Autodesk Fusion 360 part; units mm, degrees
(part 3 of 4)
sketch "草图5" plane through (-64, 0, 0) normal (-1, 0, 0) x (0, -1, 0)
  line L0 (-85, 0) -> (90, 0)
  line L1 (90, 0) -> (90, 250)
  line L2 (90, 250) -> (-85, 250)
  line L3 (-85, 250) -> (-85, 0)
  line L4 (76, 24) -> (67.3397, 19)
  line L5 (67.3397, 19) -> (67.3397, 9)
  line L6 (67.3397, 9) -> (76, 4)
  line L7 (76, 4) -> (84.6603, 9)
  line L8 (84.6603, 9) -> (84.6603, 19)
  line L9 (84.6603, 19) -> (76, 24)
  line L10 (56.6795, 24) -> (48.0192, 19)
  line L11 (48.0192, 19) -> (48.0192, 9)
  line L12 (48.0192, 9) -> (56.6795, 4)
  line L13 (56.6795, 4) -> (65.3397, 9)
  line L14 (65.3397, 9) -> (65.3397, 19)
  line L15 (65.3397, 19) -> (56.6795, 24)
  line L16 (37.359, 24) -> (28.6987, 19)
  line L17 (28.6987, 19) -> (28.6987, 9)
  line L18 (28.6987, 9) -> (37.359, 4)
  line L19 (37.359, 4) -> (46.0192, 9)
  line L20 (46.0192, 9) -> (46.0192, 19)
  line L21 (46.0192, 19) -> (37.359, 24)
  line L22 (18.0385, 24) -> (9.3782, 19)
  line L23 (9.3782, 19) -> (9.3782, 9)
  line L24 (9.3782, 9) -> (18.0385, 4)
  line L25 (18.0385, 4) -> (26.6987, 9)
  line L26 (26.6987, 9) -> (26.6987, 19)
  line L27 (26.6987, 19) -> (18.0385, 24)
  line L28 (-1.282, 24) -> (-9.9423, 19)
  line L29 (-9.9423, 19) -> (-9.9423, 9)
  line L30 (-9.9423, 9) -> (-1.282, 4)
  line L31 (-1.282, 4) -> (7.3782, 9)
  line L32 (7.3782, 9) -> (7.3782, 19)
  line L33 (7.3782, 19) -> (-1.282, 24)
  line L34 (-20.6025, 24) -> (-29.2628, 19)
  line L35 (-29.2628, 19) -> (-29.2628, 9)
  line L36 (-29.2628, 9) -> (-20.6025, 4)
  line L37 (-20.6025, 4) -> (-11.9423, 9)
  line L38 (-11.9423, 9) -> (-11.9423, 19)
  line L39 (-11.9423, 19) -> (-20.6025, 24)
  line L40 (-39.923, 24) -> (-48.5833, 19)
  line L41 (-48.5833, 19) -> (-48.5833, 9)
  line L42 (-48.5833, 9) -> (-39.923, 4)
  line L43 (-39.923, 4) -> (-31.2628, 9)
  line L44 (-31.2628, 9) -> (-31.2628, 19)
  line L45 (-31.2628, 19) -> (-39.923, 24)
  line L46 (-59.2436, 24) -> (-67.9038, 19)
  line L47 (-67.9038, 19) -> (-67.9038, 9)
  line L48 (-67.9038, 9) -> (-59.2436, 4)
  line L49 (-59.2436, 4) -> (-50.5833, 9)
  line L50 (-50.5833, 9) -> (-50.5833, 19)
  line L51 (-50.5833, 19) -> (-59.2436, 24)
  line L52 (66.3397, 40.7321) -> (57.6795, 35.7321)
  line L53 (57.6795, 35.7321) -> (57.6795, 25.7321)
  line L54 (57.6795, 25.7321) -> (66.3397, 20.7321)
  line L55 (66.3397, 20.7321) -> (75, 25.7321)
  line L56 (75, 25.7321) -> (75, 35.7321)
  line L57 (75, 35.7321) -> (66.3397, 40.7321)
  line L58 (47.0192, 40.7321) -> (38.359, 35.7321)
  line L59 (38.359, 35.7321) -> (38.359, 25.7321)
  line L60 (38.359, 25.7321) -> (47.0192, 20.7321)
  line L61 (47.0192, 20.7321) -> (55.6795, 25.7321)
  line L62 (55.6795, 25.7321) -> (55.6795, 35.7321)
  line L63 (55.6795, 35.7321) -> (47.0192, 40.7321)
  line L64 (27.6987, 40.7321) -> (19.0385, 35.7321)
  line L65 (19.0385, 35.7321) -> (19.0385, 25.7321)
  line L66 (19.0385, 25.7321) -> (27.6987, 20.7321)
  line L67 (27.6987, 20.7321) -> (36.359, 25.7321)
  line L68 (36.359, 25.7321) -> (36.359, 35.7321)
  line L69 (36.359, 35.7321) -> (27.6987, 40.7321)
  line L70 (8.3782, 40.7321) -> (-0.282, 35.7321)
  line L71 (-0.282, 35.7321) -> (-0.282, 25.7321)
  line L72 (-0.282, 25.7321) -> (8.3782, 20.7321)
  line L73 (8.3782, 20.7321) -> (17.0385, 25.7321)
  line L74 (17.0385, 25.7321) -> (17.0385, 35.7321)
  line L75 (17.0385, 35.7321) -> (8.3782, 40.7321)
  line L76 (-10.9423, 40.7321) -> (-19.6025, 35.7321)
  line L77 (-19.6025, 35.7321) -> (-19.6025, 25.7321)
  line L78 (-19.6025, 25.7321) -> (-10.9423, 20.7321)
  line L79 (-10.9423, 20.7321) -> (-2.282, 25.7321)
  line L80 (-2.282, 25.7321) -> (-2.282, 35.7321)
  line L81 (-2.282, 35.7321) -> (-10.9423, 40.7321)
  line L82 (-30.2628, 40.7321) -> (-38.923, 35.7321)
  line L83 (-38.923, 35.7321) -> (-38.923, 25.7321)
  line L84 (-38.923, 25.7321) -> (-30.2628, 20.7321)
  line L85 (-30.2628, 20.7321) -> (-21.6025, 25.7321)
  line L86 (-21.6025, 25.7321) -> (-21.6025, 35.7321)
  line L87 (-21.6025, 35.7321) -> (-30.2628, 40.7321)
  line L88 (-49.5833, 40.7321) -> (-58.2436, 35.7321)
  line L89 (-58.2436, 35.7321) -> (-58.2436, 25.7321)
  line L90 (-58.2436, 25.7321) -> (-49.5833, 20.7321)
  line L91 (-49.5833, 20.7321) -> (-40.923, 25.7321)
  line L92 (-40.923, 25.7321) -> (-40.923, 35.7321)
  line L93 (-40.923, 35.7321) -> (-49.5833, 40.7321)
  line L94 (-68.9038, 40.7321) -> (-77.5641, 35.7321)
  line L95 (-77.5641, 35.7321) -> (-77.5641, 25.7321)
  line L96 (-77.5641, 25.7321) -> (-68.9038, 20.7321)
  line L97 (-68.9038, 20.7321) -> (-60.2436, 25.7321)
  line L98 (-60.2436, 25.7321) -> (-60.2436, 35.7321)
  line L99 (-60.2436, 35.7321) -> (-68.9038, 40.7321)
  line L100 (76, 57.4641) -> (67.3397, 52.4641)
  line L101 (67.3397, 52.4641) -> (67.3397, 42.4641)
  line L102 (67.3397, 42.4641) -> (76, 37.4641)
  line L103 (76, 37.4641) -> (84.6603, 42.4641)
  line L104 (84.6603, 42.4641) -> (84.6603, 52.4641)
  line L105 (84.6603, 52.4641) -> (76, 57.4641)
  line L106 (56.6795, 57.4641) -> (48.0192, 52.4641)
  line L107 (48.0192, 52.4641) -> (48.0192, 42.4641)
  line L108 (48.0192, 42.4641) -> (56.6795, 37.4641)
  line L109 (56.6795, 37.4641) -> (65.3397, 42.4641)
  line L110 (65.3397, 42.4641) -> (65.3397, 52.4641)
  line L111 (65.3397, 52.4641) -> (56.6795, 57.4641)
  line L112 (37.359, 57.4641) -> (28.6987, 52.4641)
  line L113 (28.6987, 52.4641) -> (28.6987, 42.4641)
  line L114 (28.6987, 42.4641) -> (37.359, 37.4641)
  line L115 (37.359, 37.4641) -> (46.0192, 42.4641)
  line L116 (46.0192, 42.4641) -> (46.0192, 52.4641)
  line L117 (46.0192, 52.4641) -> (37.359, 57.4641)
  line L118 (18.0385, 57.4641) -> (9.3782, 52.4641)
  line L119 (9.3782, 52.4641) -> (9.3782, 42.4641)
  line L120 (9.3782, 42.4641) -> (18.0385, 37.4641)
  line L121 (18.0385, 37.4641) -> (26.6987, 42.4641)
  line L122 (26.6987, 42.4641) -> (26.6987, 52.4641)
  line L123 (26.6987, 52.4641) -> (18.0385, 57.4641)
  line L124 (-1.282, 57.4641) -> (-9.9423, 52.4641)
  line L125 (-9.9423, 52.4641) -> (-9.9423, 42.4641)
  line L126 (-9.9423, 42.4641) -> (-1.282, 37.4641)
  line L127 (-1.282, 37.4641) -> (7.3782, 42.4641)
  line L128 (7.3782, 42.4641) -> (7.3782, 52.4641)
  line L129 (7.3782, 52.4641) -> (-1.282, 57.4641)
  line L130 (-20.6025, 57.4641) -> (-29.2628, 52.4641)
  line L131 (-29.2628, 52.4641) -> (-29.2628, 42.4641)
  line L132 (-29.2628, 42.4641) -> (-20.6025, 37.4641)
  line L133 (-20.6025, 37.4641) -> (-11.9423, 42.4641)
  line L134 (-11.9423, 42.4641) -> (-11.9423, 52.4641)
  line L135 (-11.9423, 52.4641) -> (-20.6025, 57.4641)
  line L136 (-39.923, 57.4641) -> (-48.5833, 52.4641)
  line L137 (-48.5833, 52.4641) -> (-48.5833, 42.4641)
  line L138 (-48.5833, 42.4641) -> (-39.923, 37.4641)
  line L139 (-39.923, 37.4641) -> (-31.2628, 42.4641)
  line L140 (-31.2628, 42.4641) -> (-31.2628, 52.4641)
  line L141 (-31.2628, 52.4641) -> (-39.923, 57.4641)
  line L142 (-59.2436, 57.4641) -> (-67.9038, 52.4641)
  line L143 (-67.9038, 52.4641) -> (-67.9038, 42.4641)
  line L144 (-67.9038, 42.4641) -> (-59.2436, 37.4641)
  line L145 (-59.2436, 37.4641) -> (-50.5833, 42.4641)
  line L146 (-50.5833, 42.4641) -> (-50.5833, 52.4641)
  line L147 (-50.5833, 52.4641) -> (-59.2436, 57.4641)
  line L148 (66.3397, 74.1962) -> (57.6795, 69.1962)
  line L149 (57.6795, 69.1962) -> (57.6795, 59.1962)
  line L150 (57.6795, 59.1962) -> (66.3397, 54.1962)
  line L151 (66.3397, 54.1962) -> (75, 59.1962)
  line L152 (75, 59.1962) -> (75, 69.1962)
  line L153 (75, 69.1962) -> (66.3397, 74.1962)
  line L154 (47.0192, 74.1962) -> (38.359, 69.1962)
  line L155 (38.359, 69.1962) -> (38.359, 59.1962)
  line L156 (38.359, 59.1962) -> (47.0192, 54.1962)
  line L157 (47.0192, 54.1962) -> (55.6795, 59.1962)
  line L158 (55.6795, 59.1962) -> (55.6795, 69.1962)
  line L159 (55.6795, 69.1962) -> (47.0192, 74.1962)
  line L160 (27.6987, 74.1962) -> (19.0385, 69.1962)
  line L161 (19.0385, 69.1962) -> (19.0385, 59.1962)
  line L162 (19.0385, 59.1962) -> (27.6987, 54.1962)
  line L163 (27.6987, 54.1962) -> (36.359, 59.1962)
  line L164 (36.359, 59.1962) -> (36.359, 69.1962)
  line L165 (36.359, 69.1962) -> (27.6987, 74.1962)
  line L166 (8.3782, 74.1962) -> (-0.282, 69.1962)
  line L167 (-0.282, 69.1962) -> (-0.282, 59.1962)
  line L168 (-0.282, 59.1962) -> (8.3782, 54.1962)
  line L169 (8.3782, 54.1962) -> (17.0385, 59.1962)
  line L170 (17.0385, 59.1962) -> (17.0385, 69.1962)
  line L171 (17.0385, 69.1962) -> (8.3782, 74.1962)
  line L172 (-10.9423, 74.1962) -> (-19.6025, 69.1962)
  line L173 (-19.6025, 69.1962) -> (-19.6025, 59.1962)
  line L174 (-19.6025, 59.1962) -> (-10.9423, 54.1962)
  line L175 (-10.9423, 54.1962) -> (-2.282, 59.1962)
  line L176 (-2.282, 59.1962) -> (-2.282, 69.1962)
  line L177 (-2.282, 69.1962) -> (-10.9423, 74.1962)
  line L178 (-30.2628, 74.1962) -> (-38.923, 69.1962)
  line L179 (-38.923, 69.1962) -> (-38.923, 59.1962)
  line L180 (-38.923, 59.1962) -> (-30.2628, 54.1962)
  line L181 (-30.2628, 54.1962) -> (-21.6025, 59.1962)
  line L182 (-21.6025, 59.1962) -> (-21.6025, 69.1962)
  line L183 (-21.6025, 69.1962) -> (-30.2628, 74.1962)
  line L184 (-49.5833, 74.1962) -> (-58.2436, 69.1962)
  line L185 (-58.2436, 69.1962) -> (-58.2436, 59.1962)
  line L186 (-58.2436, 59.1962) -> (-49.5833, 54.1962)
  line L187 (-49.5833, 54.1962) -> (-40.923, 59.1962)
  line L188 (-40.923, 59.1962) -> (-40.923, 69.1962)
  line L189 (-40.923, 69.1962) -> (-49.5833, 74.1962)
  line L190 (-68.9038, 74.1962) -> (-77.5641, 69.1962)
  line L191 (-77.5641, 69.1962) -> (-77.5641, 59.1962)
  line L192 (-77.5641, 59.1962) -> (-68.9038, 54.1962)
  line L193 (-68.9038, 54.1962) -> (-60.2436, 59.1962)
  line L194 (-60.2436, 59.1962) -> (-60.2436, 69.1962)
  line L195 (-60.2436, 69.1962) -> (-68.9038, 74.1962)
  line L196 (76, 90.9282) -> (67.3397, 85.9282)
  line L197 (67.3397, 85.9282) -> (67.3397, 75.9282)
  line L198 (67.3397, 75.9282) -> (76, 70.9282)
  line L199 (76, 70.9282) -> (84.6603, 75.9282)
  line L200 (84.6603, 75.9282) -> (84.6603, 85.9282)
  line L201 (84.6603, 85.9282) -> (76, 90.9282)
  line L202 (56.6795, 90.9282) -> (48.0192, 85.9282)
  line L203 (48.0192, 85.9282) -> (48.0192, 75.9282)
  line L204 (48.0192, 75.9282) -> (56.6795, 70.9282)
  line L205 (56.6795, 70.9282) -> (65.3397, 75.9282)
  line L206 (65.3397, 75.9282) -> (65.3397, 85.9282)
  line L207 (65.3397, 85.9282) -> (56.6795, 90.9282)
  line L208 (37.359, 90.9282) -> (28.6987, 85.9282)
  line L209 (28.6987, 85.9282) -> (28.6987, 75.9282)
  line L210 (28.6987, 75.9282) -> (37.359, 70.9282)
  line L211 (37.359, 70.9282) -> (46.0192, 75.9282)
  line L212 (46.0192, 75.9282) -> (46.0192, 85.9282)
  line L213 (46.0192, 85.9282) -> (37.359, 90.9282)
  line L214 (18.0385, 90.9282) -> (9.3782, 85.9282)
  line L215 (9.3782, 85.9282) -> (9.3782, 75.9282)
  line L216 (9.3782, 75.9282) -> (18.0385, 70.9282)
  line L217 (18.0385, 70.9282) -> (26.6987, 75.9282)
  line L218 (26.6987, 75.9282) -> (26.6987, 85.9282)
  line L219 (26.6987, 85.9282) -> (18.0385, 90.9282)
  line L220 (-1.282, 90.9282) -> (-9.9423, 85.9282)
  line L221 (-9.9423, 85.9282) -> (-9.9423, 75.9282)
  line L222 (-9.9423, 75.9282) -> (-1.282, 70.9282)
  line L223 (-1.282, 70.9282) -> (7.3782, 75.9282)
  line L224 (7.3782, 75.9282) -> (7.3782, 85.9282)
  line L225 (7.3782, 85.9282) -> (-1.282, 90.9282)
  line L226 (-20.6025, 90.9282) -> (-29.2628, 85.9282)
  line L227 (-29.2628, 85.9282) -> (-29.2628, 75.9282)
  line L228 (-29.2628, 75.9282) -> (-20.6025, 70.9282)
  line L229 (-20.6025, 70.9282) -> (-11.9423, 75.9282)
  line L230 (-11.9423, 75.9282) -> (-11.9423, 85.9282)
  line L231 (-11.9423, 85.9282) -> (-20.6025, 90.9282)
  line L232 (-39.923, 90.9282) -> (-48.5833, 85.9282)
  line L233 (-48.5833, 85.9282) -> (-48.5833, 75.9282)
  line L234 (-48.5833, 75.9282) -> (-39.923, 70.9282)
  line L235 (-39.923, 70.9282) -> (-31.2628, 75.9282)
  line L236 (-31.2628, 75.9282) -> (-31.2628, 85.9282)
  line L237 (-31.2628, 85.9282) -> (-39.923, 90.9282)
  line L238 (-59.2436, 90.9282) -> (-67.9038, 85.9282)
  line L239 (-67.9038, 85.9282) -> (-67.9038, 75.9282)
  line L240 (-67.9038, 75.9282) -> (-59.2436, 70.9282)
  line L241 (-59.2436, 70.9282) -> (-50.5833, 75.9282)
  line L242 (-50.5833, 75.9282) -> (-50.5833, 85.9282)
  line L243 (-50.5833, 85.9282) -> (-59.2436, 90.9282)
  line L244 (66.3397, 107.6603) -> (57.6795, 102.6603)
  line L245 (57.6795, 102.6603) -> (57.6795, 92.6603)
  line L246 (57.6795, 92.6603) -> (66.3397, 87.6603)
  line L247 (66.3397, 87.6603) -> (75, 92.6603)
  line L248 (75, 92.6603) -> (75, 102.6603)
  line L249 (75, 102.6603) -> (66.3397, 107.6603)
  line L250 (47.0192, 107.6603) -> (38.359, 102.6603)
  line L251 (38.359, 102.6603) -> (38.359, 92.6603)
  line L252 (38.359, 92.6603) -> (47.0192, 87.6603)
  line L253 (47.0192, 87.6603) -> (55.6795, 92.6603)
  line L254 (55.6795, 92.6603) -> (55.6795, 102.6603)
  line L255 (55.6795, 102.6603) -> (47.0192, 107.6603)
  line L256 (27.6987, 107.6603) -> (19.0385, 102.6603)
  line L257 (19.0385, 102.6603) -> (19.0385, 92.6603)
  line L258 (19.0385, 92.6603) -> (27.6987, 87.6603)
  line L259 (27.6987, 87.6603) -> (36.359, 92.6603)
  line L260 (36.359, 92.6603) -> (36.359, 102.6603)
  line L261 (36.359, 102.6603) -> (27.6987, 107.6603)
  line L262 (8.3782, 107.6603) -> (-0.282, 102.6603)
  line L263 (-0.282, 102.6603) -> (-0.282, 92.6603)
  line L264 (-0.282, 92.6603) -> (8.3782, 87.6603)
  line L265 (8.3782, 87.6603) -> (17.0385, 92.6603)
  line L266 (17.0385, 92.6603) -> (17.0385, 102.6603)
  line L267 (17.0385, 102.6603) -> (8.3782, 107.6603)
  line L268 (-10.9423, 107.6603) -> (-19.6025, 102.6603)
  line L269 (-19.6025, 102.6603) -> (-19.6025, 92.6603)
  line L270 (-19.6025, 92.6603) -> (-10.9423, 87.6603)
  line L271 (-10.9423, 87.6603) -> (-2.282, 92.6603)
  line L272 (-2.282, 92.6603) -> (-2.282, 102.6603)
  line L273 (-2.282, 102.6603) -> (-10.9423, 107.6603)
  line L274 (-30.2628, 107.6603) -> (-38.923, 102.6603)
  line L275 (-38.923, 102.6603) -> (-38.923, 92.6603)
  line L276 (-38.923, 92.6603) -> (-30.2628, 87.6603)
  line L277 (-30.2628, 87.6603) -> (-21.6025, 92.6603)
  line L278 (-21.6025, 92.6603) -> (-21.6025, 102.6603)
  line L279 (-21.6025, 102.6603) -> (-30.2628, 107.6603)
  line L280 (-49.5833, 107.6603) -> (-58.2436, 102.6603)
  line L281 (-58.2436, 102.6603) -> (-58.2436, 92.6603)
  line L282 (-58.2436, 92.6603) -> (-49.5833, 87.6603)
  line L283 (-49.5833, 87.6603) -> (-40.923, 92.6603)
  line L284 (-40.923, 92.6603) -> (-40.923, 102.6603)
  line L285 (-40.923, 102.6603) -> (-49.5833, 107.6603)
  line L286 (-68.9038, 107.6603) -> (-77.5641, 102.6603)
  line L287 (-77.5641, 102.6603) -> (-77.5641, 92.6603)
  line L288 (-77.5641, 92.6603) -> (-68.9038, 87.6603)
  line L289 (-68.9038, 87.6603) -> (-60.2436, 92.6603)
  line L290 (-60.2436, 92.6603) -> (-60.2436, 102.6603)
  line L291 (-60.2436, 102.6603) -> (-68.9038, 107.6603)
  line L292 (76, 124.3923) -> (67.3397, 119.3923)
  line L293 (67.3397, 119.3923) -> (67.3397, 109.3923)
  line L294 (67.3397, 109.3923) -> (76, 104.3923)
  line L295 (76, 104.3923) -> (84.6603, 109.3923)
  line L296 (84.6603, 109.3923) -> (84.6603, 119.3923)
  line L297 (84.6603, 119.3923) -> (76, 124.3923)
  line L298 (56.6795, 124.3923) -> (48.0192, 119.3923)
  line L299 (48.0192, 119.3923) -> (48.0192, 109.3923)
  line L300 (48.0192, 109.3923) -> (56.6795, 104.3923)
  line L301 (56.6795, 104.3923) -> (65.3397, 109.3923)
  line L302 (65.3397, 109.3923) -> (65.3397, 119.3923)
  line L303 (65.3397, 119.3923) -> (56.6795, 124.3923)
  line L304 (37.359, 124.3923) -> (28.6987, 119.3923)
  line L305 (28.6987, 119.3923) -> (28.6987, 109.3923)
  line L306 (28.6987, 109.3923) -> (37.359, 104.3923)
  line L307 (37.359, 104.3923) -> (46.0192, 109.3923)
  line L308 (46.0192, 109.3923) -> (46.0192, 119.3923)
  line L309 (46.0192, 119.3923) -> (37.359, 124.3923)
  line L310 (18.0385, 124.3923) -> (9.3782, 119.3923)
  line L311 (9.3782, 119.3923) -> (9.3782, 109.3923)
  line L312 (9.3782, 109.3923) -> (18.0385, 104.3923)
  line L313 (18.0385, 104.3923) -> (26.6987, 109.3923)
  line L314 (26.6987, 109.3923) -> (26.6987, 119.3923)
  line L315 (26.6987, 119.3923) -> (18.0385, 124.3923)
  line L316 (-1.282, 124.3923) -> (-9.9423, 119.3923)
  line L317 (-9.9423, 119.3923) -> (-9.9423, 109.3923)
  line L318 (-9.9423, 109.3923) -> (-1.282, 104.3923)
  line L319 (-1.282, 104.3923) -> (7.3782, 109.3923)
  line L320 (7.3782, 109.3923) -> (7.3782, 119.3923)
  line L321 (7.3782, 119.3923) -> (-1.282, 124.3923)
  line L322 (-20.6025, 124.3923) -> (-29.2628, 119.3923)
  line L323 (-29.2628, 119.3923) -> (-29.2628, 109.3923)
  line L324 (-29.2628, 109.3923) -> (-20.6025, 104.3923)
  line L325 (-20.6025, 104.3923) -> (-11.9423, 109.3923)
  line L326 (-11.9423, 109.3923) -> (-11.9423, 119.3923)
  line L327 (-11.9423, 119.3923) -> (-20.6025, 124.3923)
  line L328 (-39.923, 124.3923) -> (-48.5833, 119.3923)
  line L329 (-48.5833, 119.3923) -> (-48.5833, 109.3923)
  line L330 (-48.5833, 109.3923) -> (-39.923, 104.3923)
  line L331 (-39.923, 104.3923) -> (-31.2628, 109.3923)
  line L332 (-31.2628, 109.3923) -> (-31.2628, 119.3923)
  line L333 (-31.2628, 119.3923) -> (-39.923, 124.3923)
  line L334 (-59.2436, 124.3923) -> (-67.9038, 119.3923)
  line L335 (-67.9038, 119.3923) -> (-67.9038, 109.3923)
  line L336 (-67.9038, 109.3923) -> (-59.2436, 104.3923)
  line L337 (-59.2436, 104.3923) -> (-50.5833, 109.3923)
  line L338 (-50.5833, 109.3923) -> (-50.5833, 119.3923)
  line L339 (-50.5833, 119.3923) -> (-59.2436, 124.3923)
  line L340 (66.3397, 141.1244) -> (57.6795, 136.1244)
  line L341 (57.6795, 136.1244) -> (57.6795, 126.1244)
  line L342 (57.6795, 126.1244) -> (66.3397, 121.1244)
  line L343 (66.3397, 121.1244) -> (75, 126.1244)
  line L344 (75, 126.1244) -> (75, 136.1244)
  line L345 (75, 136.1244) -> (66.3397, 141.1244)
  line L346 (47.0192, 141.1244) -> (38.359, 136.1244)
  line L347 (38.359, 136.1244) -> (38.359, 126.1244)
  line L348 (38.359, 126.1244) -> (47.0192, 121.1244)
  line L349 (47.0192, 121.1244) -> (55.6795, 126.1244)
  line L350 (55.6795, 126.1244) -> (55.6795, 136.1244)
  line L351 (55.6795, 136.1244) -> (47.0192, 141.1244)
  line L352 (27.6987, 141.1244) -> (19.0385, 136.1244)
  line L353 (19.0385, 136.1244) -> (19.0385, 126.1244)
  line L354 (19.0385, 126.1244) -> (27.6987, 121.1244)
  line L355 (27.6987, 121.1244) -> (36.359, 126.1244)
  line L356 (36.359, 126.1244) -> (36.359, 136.1244)
  line L357 (36.359, 136.1244) -> (27.6987, 141.1244)
  line L358 (8.3782, 141.1244) -> (-0.282, 136.1244)
  line L359 (-0.282, 136.1244) -> (-0.282, 126.1244)
  line L360 (-0.282, 126.1244) -> (8.3782, 121.1244)
  line L361 (8.3782, 121.1244) -> (17.0385, 126.1244)
  line L362 (17.0385, 126.1244) -> (17.0385, 136.1244)
  line L363 (17.0385, 136.1244) -> (8.3782, 141.1244)
  line L364 (-10.9423, 141.1244) -> (-19.6025, 136.1244)
  line L365 (-19.6025, 136.1244) -> (-19.6025, 126.1244)
  line L366 (-19.6025, 126.1244) -> (-10.9423, 121.1244)
  line L367 (-10.9423, 121.1244) -> (-2.282, 126.1244)
  line L368 (-2.282, 126.1244) -> (-2.282, 136.1244)
  line L369 (-2.282, 136.1244) -> (-10.9423, 141.1244)
  line L370 (-30.2628, 141.1244) -> (-38.923, 136.1244)
  line L371 (-38.923, 136.1244) -> (-38.923, 126.1244)
  line L372 (-38.923, 126.1244) -> (-30.2628, 121.1244)
  line L373 (-30.2628, 121.1244) -> (-21.6025, 126.1244)
  line L374 (-21.6025, 126.1244) -> (-21.6025, 136.1244)
  line L375 (-21.6025, 136.1244) -> (-30.2628, 141.1244)
  line L376 (-49.5833, 141.1244) -> (-58.2436, 136.1244)
  line L377 (-58.2436, 136.1244) -> (-58.2436, 126.1244)
  line L378 (-58.2436, 126.1244) -> (-49.5833, 121.1244)
  line L379 (-49.5833, 121.1244) -> (-40.923, 126.1244)
  line L380 (-40.923, 126.1244) -> (-40.923, 136.1244)
  line L381 (-40.923, 136.1244) -> (-49.5833, 141.1244)
  line L382 (-68.9038, 141.1244) -> (-77.5641, 136.1244)
  line L383 (-77.5641, 136.1244) -> (-77.5641, 126.1244)
  line L384 (-77.5641, 126.1244) -> (-68.9038, 121.1244)
  line L385 (-68.9038, 121.1244) -> (-60.2436, 126.1244)
  line L386 (-60.2436, 126.1244) -> (-60.2436, 136.1244)
  line L387 (-60.2436, 136.1244) -> (-68.9038, 141.1244)
  line L388 (76, 157.8564) -> (67.3397, 152.8564)
  line L389 (67.3397, 152.8564) -> (67.3397, 142.8564)
  line L390 (67.3397, 142.8564) -> (76, 137.8564)
  line L391 (76, 137.8564) -> (84.6603, 142.8564)
  line L392 (84.6603, 142.8564) -> (84.6603, 152.8564)
  line L393 (84.6603, 152.8564) -> (76, 157.8564)
  line L394 (56.6795, 157.8564) -> (48.0192, 152.8564)
  line L395 (48.0192, 152.8564) -> (48.0192, 142.8564)
  line L396 (48.0192, 142.8564) -> (56.6795, 137.8564)
  line L397 (56.6795, 137.8564) -> (65.3397, 142.8564)
  line L398 (65.3397, 142.8564) -> (65.3397, 152.8564)
  line L399 (65.3397, 152.8564) -> (56.6795, 157.8564)
  line L400 (37.359, 157.8564) -> (28.6987, 152.8564)
  line L401 (28.6987, 152.8564) -> (28.6987, 142.8564)
  line L402 (28.6987, 142.8564) -> (37.359, 137.8564)
  line L403 (37.359, 137.8564) -> (46.0192, 142.8564)
  line L404 (46.0192, 142.8564) -> (46.0192, 152.8564)
  line L405 (46.0192, 152.8564) -> (37.359, 157.8564)
  line L406 (18.0385, 157.8564) -> (9.3782, 152.8564)
  line L407 (9.3782, 152.8564) -> (9.3782, 142.8564)
  line L408 (9.3782, 142.8564) -> (18.0385, 137.8564)
  line L409 (18.0385, 137.8564) -> (26.6987, 142.8564)
  line L410 (26.6987, 142.8564) -> (26.6987, 152.8564)
  line L411 (26.6987, 152.8564) -> (18.0385, 157.8564)
  line L412 (-1.282, 157.8564) -> (-9.9423, 152.8564)
  line L413 (-9.9423, 152.8564) -> (-9.9423, 142.8564)
  line L414 (-9.9423, 142.8564) -> (-1.282, 137.8564)
  line L415 (-1.282, 137.8564) -> (7.3782, 142.8564)
  line L416 (7.3782, 142.8564) -> (7.3782, 152.8564)
  line L417 (7.3782, 152.8564) -> (-1.282, 157.8564)
  line L418 (-20.6025, 157.8564) -> (-29.2628, 152.8564)
  line L419 (-29.2628, 152.8564) -> (-29.2628, 142.8564)
  line L420 (-29.2628, 142.8564) -> (-20.6025, 137.8564)
  line L421 (-20.6025, 137.8564) -> (-11.9423, 142.8564)
  line L422 (-11.9423, 142.8564) -> (-11.9423, 152.8564)
  line L423 (-11.9423, 152.8564) -> (-20.6025, 157.8564)
  line L424 (-39.923, 157.8564) -> (-48.5833, 152.8564)
  line L425 (-48.5833, 152.8564) -> (-48.5833, 142.8564)
  line L426 (-48.5833, 142.8564) -> (-39.923, 137.8564)
  line L427 (-39.923, 137.8564) -> (-31.2628, 142.8564)
  line L428 (-31.2628, 142.8564) -> (-31.2628, 152.8564)
  line L429 (-31.2628, 152.8564) -> (-39.923, 157.8564)
  line L430 (-59.2436, 157.8564) -> (-67.9038, 152.8564)
  line L431 (-67.9038, 152.8564) -> (-67.9038, 142.8564)
  line L432 (-67.9038, 142.8564) -> (-59.2436, 137.8564)
  line L433 (-59.2436, 137.8564) -> (-50.5833, 142.8564)
  line L434 (-50.5833, 142.8564) -> (-50.5833, 152.8564)
  line L435 (-50.5833, 152.8564) -> (-59.2436, 157.8564)
  line L436 (66.3397, 174.5885) -> (57.6795, 169.5885)
  line L437 (57.6795, 169.5885) -> (57.6795, 159.5885)
  line L438 (57.6795, 159.5885) -> (66.3397, 154.5885)
  line L439 (66.3397, 154.5885) -> (75, 159.5885)
  line L440 (75, 159.5885) -> (75, 169.5885)
  line L441 (75, 169.5885) -> (66.3397, 174.5885)
  line L442 (47.0192, 174.5885) -> (38.359, 169.5885)
  line L443 (38.359, 169.5885) -> (38.359, 159.5885)
  line L444 (38.359, 159.5885) -> (47.0192, 154.5885)
  line L445 (47.0192, 154.5885) -> (55.6795, 159.5885)
  line L446 (55.6795, 159.5885) -> (55.6795, 169.5885)
  line L447 (55.6795, 169.5885) -> (47.0192, 174.5885)
  line L448 (27.6987, 174.5885) -> (19.0385, 169.5885)
  line L449 (19.0385, 169.5885) -> (19.0385, 159.5885)
  line L450 (19.0385, 159.5885) -> (27.6987, 154.5885)
  line L451 (27.6987, 154.5885) -> (36.359, 159.5885)
  line L452 (36.359, 159.5885) -> (36.359, 169.5885)
  line L453 (36.359, 169.5885) -> (27.6987, 174.5885)
  line L454 (8.3782, 174.5885) -> (-0.282, 169.5885)
  line L455 (-0.282, 169.5885) -> (-0.282, 159.5885)
  line L456 (-0.282, 159.5885) -> (8.3782, 154.5885)
  line L457 (8.3782, 154.5885) -> (17.0385, 159.5885)
  line L458 (17.0385, 159.5885) -> (17.0385, 169.5885)
  line L459 (17.0385, 169.5885) -> (8.3782, 174.5885)
  line L460 (-10.9423, 174.5885) -> (-19.6025, 169.5885)
  line L461 (-19.6025, 169.5885) -> (-19.6025, 159.5885)
  line L462 (-19.6025, 159.5885) -> (-10.9423, 154.5885)
  line L463 (-10.9423, 154.5885) -> (-2.282, 159.5885)
  line L464 (-2.282, 159.5885) -> (-2.282, 169.5885)
  line L465 (-2.282, 169.5885) -> (-10.9423, 174.5885)
  line L466 (-30.2628, 174.5885) -> (-38.923, 169.5885)
  line L467 (-38.923, 169.5885) -> (-38.923, 159.5885)
  line L468 (-38.923, 159.5885) -> (-30.2628, 154.5885)
  line L469 (-30.2628, 154.5885) -> (-21.6025, 159.5885)
  line L470 (-21.6025, 159.5885) -> (-21.6025, 169.5885)
  line L471 (-21.6025, 169.5885) -> (-30.2628, 174.5885)
  line L472 (-49.5833, 174.5885) -> (-58.2436, 169.5885)
  line L473 (-58.2436, 169.5885) -> (-58.2436, 159.5885)
  line L474 (-58.2436, 159.5885) -> (-49.5833, 154.5885)
  line L475 (-49.5833, 154.5885) -> (-40.923, 159.5885)
  line L476 (-40.923, 159.5885) -> (-40.923, 169.5885)
  line L477 (-40.923, 169.5885) -> (-49.5833, 174.5885)
  line L478 (-68.9038, 174.5885) -> (-77.5641, 169.5885)
  line L479 (-77.5641, 169.5885) -> (-77.5641, 159.5885)
  line L480 (-77.5641, 159.5885) -> (-68.9038, 154.5885)
  line L481 (-68.9038, 154.5885) -> (-60.2436, 159.5885)
  line L482 (-60.2436, 159.5885) -> (-60.2436, 169.5885)
  line L483 (-60.2436, 169.5885) -> (-68.9038, 174.5885)
  line L484 (76, 191.3205) -> (67.3397, 186.3205)
  line L485 (67.3397, 186.3205) -> (67.3397, 176.3205)
  line L486 (67.3397, 176.3205) -> (76, 171.3205)
  line L487 (76, 171.3205) -> (84.6603, 176.3205)
  line L488 (84.6603, 176.3205) -> (84.6603, 186.3205)
  line L489 (84.6603, 186.3205) -> (76, 191.3205)
  line L490 (56.6795, 191.3205) -> (48.0192, 186.3205)
  line L491 (48.0192, 186.3205) -> (48.0192, 176.3205)
  line L492 (48.0192, 176.3205) -> (56.6795, 171.3205)
  line L493 (56.6795, 171.3205) -> (65.3397, 176.3205)
  line L494 (65.3397, 176.3205) -> (65.3397, 186.3205)
  line L495 (65.3397, 186.3205) -> (56.6795, 191.3205)
  line L496 (37.359, 191.3205) -> (28.6987, 186.3205)
  line L497 (28.6987, 186.3205) -> (28.6987, 176.3205)
  line L498 (28.6987, 176.3205) -> (37.359, 171.3205)
  line L499 (37.359, 171.3205) -> (46.0192, 176.3205)
  line L500 (46.0192, 176.3205) -> (46.0192, 186.3205)
  line L501 (46.0192, 186.3205) -> (37.359, 191.3205)
  line L502 (18.0385, 191.3205) -> (9.3782, 186.3205)
  line L503 (9.3782, 186.3205) -> (9.3782, 176.3205)
  line L504 (9.3782, 176.3205) -> (18.0385, 171.3205)
  line L505 (18.0385, 171.3205) -> (26.6987, 176.3205)
  line L506 (26.6987, 176.3205) -> (26.6987, 186.3205)
  line L507 (26.6987, 186.3205) -> (18.0385, 191.3205)
  line L508 (-1.282, 191.3205) -> (-9.9423, 186.3205)
  line L509 (-9.9423, 186.3205) -> (-9.9423, 176.3205)
  line L510 (-9.9423, 176.3205) -> (-1.282, 171.3205)
  line L511 (-1.282, 171.3205) -> (7.3782, 176.3205)
  line L512 (7.3782, 176.3205) -> (7.3782, 186.3205)
  line L513 (7.3782, 186.3205) -> (-1.282, 191.3205)
  line L514 (-20.6025, 191.3205) -> (-29.2628, 186.3205)
  line L515 (-29.2628, 186.3205) -> (-29.2628, 176.3205)
  line L516 (-29.2628, 176.3205) -> (-20.6025, 171.3205)
  line L517 (-20.6025, 171.3205) -> (-11.9423, 176.3205)
  line L518 (-11.9423, 176.3205) -> (-11.9423, 186.3205)
  line L519 (-11.9423, 186.3205) -> (-20.6025, 191.3205)
  line L520 (-39.923, 191.3205) -> (-48.5833, 186.3205)
  line L521 (-48.5833, 186.3205) -> (-48.5833, 176.3205)
  line L522 (-48.5833, 176.3205) -> (-39.923, 171.3205)
  line L523 (-39.923, 171.3205) -> (-31.2628, 176.3205)
  line L524 (-31.2628, 176.3205) -> (-31.2628, 186.3205)
  line L525 (-31.2628, 186.3205) -> (-39.923, 191.3205)
  line L526 (-59.2436, 191.3205) -> (-67.9038, 186.3205)
  line L527 (-67.9038, 186.3205) -> (-67.9038, 176.3205)
  line L528 (-67.9038, 176.3205) -> (-59.2436, 171.3205)
  line L529 (-59.2436, 171.3205) -> (-50.5833, 176.3205)
  line L530 (-50.5833, 176.3205) -> (-50.5833, 186.3205)
  line L531 (-50.5833, 186.3205) -> (-59.2436, 191.3205)
  line L532 (66.3397, 208.0526) -> (57.6795, 203.0526)
  line L533 (57.6795, 203.0526) -> (57.6795, 193.0526)
  line L534 (57.6795, 193.0526) -> (66.3397, 188.0526)
  line L535 (66.3397, 188.0526) -> (75, 193.0526)
  line L536 (75, 193.0526) -> (75, 203.0526)
  line L537 (75, 203.0526) -> (66.3397, 208.0526)
  line L538 (47.0192, 208.0526) -> (38.359, 203.0526)
  line L539 (38.359, 203.0526) -> (38.359, 193.0526)
  line L540 (38.359, 193.0526) -> (47.0192, 188.0526)
  line L541 (47.0192, 188.0526) -> (55.6795, 193.0526)
  line L542 (55.6795, 193.0526) -> (55.6795, 203.0526)
  line L543 (55.6795, 203.0526) -> (47.0192, 208.0526)
  line L544 (27.6987, 208.0526) -> (19.0385, 203.0526)
  line L545 (19.0385, 203.0526) -> (19.0385, 193.0526)
  line L546 (19.0385, 193.0526) -> (27.6987, 188.0526)
  line L547 (27.6987, 188.0526) -> (36.359, 193.0526)
  line L548 (36.359, 193.0526) -> (36.359, 203.0526)
  line L549 (36.359, 203.0526) -> (27.6987, 208.0526)
  line L550 (8.3782, 208.0526) -> (-0.282, 203.0526)
  line L551 (-0.282, 203.0526) -> (-0.282, 193.0526)
  line L552 (-0.282, 193.0526) -> (8.3782, 188.0526)
  line L553 (8.3782, 188.0526) -> (17.0385, 193.0526)
  line L554 (17.0385, 193.0526) -> (17.0385, 203.0526)
  line L555 (17.0385, 203.0526) -> (8.3782, 208.0526)
  line L556 (-10.9423, 208.0526) -> (-19.6025, 203.0526)
  line L557 (-19.6025, 203.0526) -> (-19.6025, 193.0526)
  line L558 (-19.6025, 193.0526) -> (-10.9423, 188.0526)
  line L559 (-10.9423, 188.0526) -> (-2.282, 193.0526)
  line L560 (-2.282, 193.0526) -> (-2.282, 203.0526)
  line L561 (-2.282, 203.0526) -> (-10.9423, 208.0526)
  line L562 (-30.2628, 208.0526) -> (-38.923, 203.0526)
  line L563 (-38.923, 203.0526) -> (-38.923, 193.0526)
  line L564 (-38.923, 193.0526) -> (-30.2628, 188.0526)
  line L565 (-30.2628, 188.0526) -> (-21.6025, 193.0526)
  line L566 (-21.6025, 193.0526) -> (-21.6025, 203.0526)
  line L567 (-21.6025, 203.0526) -> (-30.2628, 208.0526)
  line L568 (-49.5833, 208.0526) -> (-58.2436, 203.0526)
  line L569 (-58.2436, 203.0526) -> (-58.2436, 193.0526)
  line L570 (-58.2436, 193.0526) -> (-49.5833, 188.0526)
  line L571 (-49.5833, 188.0526) -> (-40.923, 193.0526)
  line L572 (-40.923, 193.0526) -> (-40.923, 203.0526)
  line L573 (-40.923, 203.0526) -> (-49.5833, 208.0526)
  line L574 (-68.9038, 208.0526) -> (-77.5641, 203.0526)
  line L575 (-77.5641, 203.0526) -> (-77.5641, 193.0526)
  line L576 (-77.5641, 193.0526) -> (-68.9038, 188.0526)
  line L577 (-68.9038, 188.0526) -> (-60.2436, 193.0526)
  line L578 (-60.2436, 193.0526) -> (-60.2436, 203.0526)
  line L579 (-60.2436, 203.0526) -> (-68.9038, 208.0526)
  line L580 (76, 224.7846) -> (67.3397, 219.7846)
  line L581 (67.3397, 219.7846) -> (67.3397, 209.7846)
  line L582 (67.3397, 209.7846) -> (76, 204.7846)
  line L583 (76, 204.7846) -> (84.6603, 209.7846)
  line L584 (84.6603, 209.7846) -> (84.6603, 219.7846)
  line L585 (84.6603, 219.7846) -> (76, 224.7846)
  line L586 (56.6795, 224.7846) -> (48.0192, 219.7846)
  line L587 (48.0192, 219.7846) -> (48.0192, 209.7846)
  line L588 (48.0192, 209.7846) -> (56.6795, 204.7846)
  line L589 (56.6795, 204.7846) -> (65.3397, 209.7846)
  line L590 (65.3397, 209.7846) -> (65.3397, 219.7846)
  line L591 (65.3397, 219.7846) -> (56.6795, 224.7846)
  line L592 (37.359, 224.7846) -> (28.6987, 219.7846)
  line L593 (28.6987, 219.7846) -> (28.6987, 209.7846)
  line L594 (28.6987, 209.7846) -> (37.359, 204.7846)
  line L595 (37.359, 204.7846) -> (46.0192, 209.7846)
  line L596 (46.0192, 209.7846) -> (46.0192, 219.7846)
  line L597 (46.0192, 219.7846) -> (37.359, 224.7846)
  line L598 (18.0385, 224.7846) -> (9.3782, 219.7846)
  line L599 (9.3782, 219.7846) -> (9.3782, 209.7846)
  line L600 (9.3782, 209.7846) -> (18.0385, 204.7846)
  line L601 (18.0385, 204.7846) -> (26.6987, 209.7846)
  line L602 (26.6987, 209.7846) -> (26.6987, 219.7846)
  line L603 (26.6987, 219.7846) -> (18.0385, 224.7846)
  line L604 (-1.282, 224.7846) -> (-9.9423, 219.7846)
  line L605 (-9.9423, 219.7846) -> (-9.9423, 209.7846)
  line L606 (-9.9423, 209.7846) -> (-1.282, 204.7846)
  line L607 (-1.282, 204.7846) -> (7.3782, 209.7846)
  line L608 (7.3782, 209.7846) -> (7.3782, 219.7846)
  line L609 (7.3782, 219.7846) -> (-1.282, 224.7846)
  line L610 (-20.6025, 224.7846) -> (-29.2628, 219.7846)
  line L611 (-29.2628, 219.7846) -> (-29.2628, 209.7846)
  line L612 (-29.2628, 209.7846) -> (-20.6025, 204.7846)
  line L613 (-20.6025, 204.7846) -> (-11.9423, 209.7846)
  line L614 (-11.9423, 209.7846) -> (-11.9423, 219.7846)
  line L615 (-11.9423, 219.7846) -> (-20.6025, 224.7846)
  line L616 (-39.923, 224.7846) -> (-48.5833, 219.7846)
  line L617 (-48.5833, 219.7846) -> (-48.5833, 209.7846)
  line L618 (-48.5833, 209.7846) -> (-39.923, 204.7846)
  line L619 (-39.923, 204.7846) -> (-31.2628, 209.7846)
  line L620 (-31.2628, 209.7846) -> (-31.2628, 219.7846)
  line L621 (-31.2628, 219.7846) -> (-39.923, 224.7846)
  line L622 (-59.2436, 224.7846) -> (-67.9038, 219.7846)
  line L623 (-67.9038, 219.7846) -> (-67.9038, 209.7846)
  line L624 (-67.9038, 209.7846) -> (-59.2436, 204.7846)
  line L625 (-59.2436, 204.7846) -> (-50.5833, 209.7846)
  line L626 (-50.5833, 209.7846) -> (-50.5833, 219.7846)
  line L627 (-50.5833, 219.7846) -> (-59.2436, 224.7846)
  line L628 (66.3397, 241.5167) -> (57.6795, 236.5167)
  line L629 (57.6795, 236.5167) -> (57.6795, 226.5167)
  line L630 (57.6795, 226.5167) -> (66.3397, 221.5167)
  line L631 (66.3397, 221.5167) -> (75, 226.5167)
  line L632 (75, 226.5167) -> (75, 236.5167)
  line L633 (75, 236.5167) -> (66.3397, 241.5167)
  line L634 (47.0192, 241.5167) -> (38.359, 236.5167)
  line L635 (38.359, 236.5167) -> (38.359, 226.5167)
  line L636 (38.359, 226.5167) -> (47.0192, 221.5167)
  line L637 (47.0192, 221.5167) -> (55.6795, 226.5167)
  line L638 (55.6795, 226.5167) -> (55.6795, 236.5167)
  line L639 (55.6795, 236.5167) -> (47.0192, 241.5167)
  line L640 (27.6987, 241.5167) -> (19.0385, 236.5167)
  line L641 (19.0385, 236.5167) -> (19.0385, 226.5167)
  line L642 (19.0385, 226.5167) -> (27.6987, 221.5167)
  line L643 (27.6987, 221.5167) -> (36.359, 226.5167)
  line L644 (36.359, 226.5167) -> (36.359, 236.5167)
  line L645 (36.359, 236.5167) -> (27.6987, 241.5167)
  line L646 (8.3782, 241.5167) -> (-0.282, 236.5167)
  line L647 (-0.282, 236.5167) -> (-0.282, 226.5167)
  line L648 (-0.282, 226.5167) -> (8.3782, 221.5167)
  line L649 (8.3782, 221.5167) -> (17.0385, 226.5167)
  line L650 (17.0385, 226.5167) -> (17.0385, 236.5167)
  line L651 (17.0385, 236.5167) -> (8.3782, 241.5167)
  line L652 (-10.9423, 241.5167) -> (-19.6025, 236.5167)
  line L653 (-19.6025, 236.5167) -> (-19.6025, 226.5167)
  line L654 (-19.6025, 226.5167) -> (-10.9423, 221.5167)
  line L655 (-10.9423, 221.5167) -> (-2.282, 226.5167)
  line L656 (-2.282, 226.5167) -> (-2.282, 236.5167)
  line L657 (-2.282, 236.5167) -> (-10.9423, 241.5167)
  line L658 (-30.2628, 241.5167) -> (-38.923, 236.5167)
  line L659 (-38.923, 236.5167) -> (-38.923, 226.5167)
  line L660 (-38.923, 226.5167) -> (-30.2628, 221.5167)
  line L661 (-30.2628, 221.5167) -> (-21.6025, 226.5167)
  line L662 (-21.6025, 226.5167) -> (-21.6025, 236.5167)
  line L663 (-21.6025, 236.5167) -> (-30.2628, 241.5167)
  line L664 (-49.5833, 241.5167) -> (-58.2436, 236.5167)
  line L665 (-58.2436, 236.5167) -> (-58.2436, 226.5167)
  line L666 (-58.2436, 226.5167) -> (-49.5833, 221.5167)
  line L667 (-49.5833, 221.5167) -> (-40.923, 226.5167)
  line L668 (-40.923, 226.5167) -> (-40.923, 236.5167)
  line L669 (-40.923, 236.5167) -> (-49.5833, 241.5167)
  line L670 (-68.9038, 241.5167) -> (-77.5641, 236.5167)
  line L671 (-77.5641, 236.5167) -> (-77.5641, 226.5167)
  line L672 (-77.5641, 226.5167) -> (-68.9038, 221.5167)
  line L673 (-68.9038, 221.5167) -> (-60.2436, 226.5167)
  line L674 (-60.2436, 226.5167) -> (-60.2436, 236.5167)
  line L675 (-60.2436, 236.5167) -> (-68.9038, 241.5167)
extrude "拉伸5" cut sketch "草图5" against normal blind 4 contours L4 L5 L6 L7 L8 L9 | L10 L11 L12 L13 L14 L15 | L16 L17 L18 L19 L20 L21 | L22 L23 L24 L25 L26 L27 | L28 L29 L30 L31 L32 L33 | L34 L35 L36 L37 L38 L39 | L40 L41 L42 L43 L44 L45 | L46 L47 L48 L49 L50 L51 | L52 L53 L54 L55 L56 L57 | L58 L59 L60 L61 L62 L63 | L64 L65 L66 L67 L68 L69 | L70 L71 L72 L73 L74 L75 | L76 L77 L78 L79 L80 L81 | L82 L83 L84 L85 L86 L87 | L88 L89 L90 L91 L92 L93 | L94 L95 L96 L97 L98 L99 | L100 L101 L102 L103 L104 L105 | L106 L107 L108 L109 L110 L111 | L112 L113 L114 L115 L116 L117 | L118 L119 L120 L121 L122 L123 | L124 L125 L126 L127 L128 L129 | L130 L131 L132 L133 L134 L135 | L136 L137 L138 L139 L140 L141 | L142 L143 L144 L145 L146 L147 | L148 L149 L150 L151 L152 L153 | L154 L155 L156 L157 L158 L159 | L160 L161 L162 L163 L164 L165 | L166 L167 L168 L169 L170 L171 | L172 L173 L174 L175 L176 L177 | L178 L179 L180 L181 L182 L183 | L184 L185 L186 L187 L188 L189 | L190 L191 L192 L193 L194 L195 | L196 L197 L198 L199 L200 L201 | L202 L203 L204 L205 L206 L207 | L208 L209 L210 L211 L212 L213 | L214 L215 L216 L217 L218 L219 | L220 L221 L222 L223 L224 L225 | L226 L227 L228 L229 L230 L231 | L232 L233 L234 L235 L236 L237 | L238 L239 L240 L241 L242 L243 | L244 L245 L246 L247 L248 L249 | L250 L251 L252 L253 L254 L255 | L256 L257 L258 L259 L260 L261 | L262 L263 L264 L265 L266 L267 | L268 L269 L270 L271 L272 L273 | L274 L275 L276 L277 L278 L279 | L280 L281 L282 L283 L284 L285 | L286 L287 L288 L289 L290 L291 | L292 L293 L294 L295 L296 L297 | L298 L299 L300 L301 L302 L303 | L304 L305 L306 L307 L308 L309 | L310 L311 L312 L313 L314 L315 | L316 L317 L318 L319 L320 L321 | L322 L323 L324 L325 L326 L327 | L328 L329 L330 L331 L332 L333 | L334 L335 L336 L337 L338 L339 | L340 L341 L342 L343 L344 L345 | L346 L347 L348 L349 L350 L351 | L352 L353 L354 L355 L356 L357 | L358 L359 L360 L361 L362 L363 | L364 L365 L366 L367 L368 L369 | L370 L371 L372 L373 L374 L375 | L376 L377 L378 L379 L380 L381 | L382 L383 L384 L385 L386 L387 | L388 L389 L390 L391 L392 L393 | L394 L395 L396 L397 L398 L399 | L400 L401 L402 L403 L404 L405 | L406 L407 L408 L409 L410 L411 | L412 L413 L414 L415 L416 L417 | L418 L419 L420 L421 L422 L423 | L424 L425 L426 L427 L428 L429 | L430 L431 L432 L433 L434 L435 | L436 L437 L438 L439 L440 L441 | L442 L443 L444 L445 L446 L447 | L448 L449 L450 L451 L452 L453 | L454 L455 L456 L457 L458 L459 | L460 L461 L462 L463 L464 L465 | L466 L467 L468 L469 L470 L471 | L472 L473 L474 L475 L476 L477 | L478 L479 L480 L481 L482 L483 | L484 L485 L486 L487 L488 L489 | L490 L491 L492 L493 L494 L495 | L496 L497 L498 L499 L500 L501 | L502 L503 L504 L505 L506 L507 | L508 L509 L510 L511 L512 L513 | L514 L515 L516 L517 L518 L519 | L520 L521 L522 L523 L524 L525 | L526 L527 L528 L529 L530 L531 | L532 L533 L534 L535 L536 L537 | L538 L539 L540 L541 L542 L543 | L544 L545 L546 L547 L548 L549 | L550 L551 L552 L553 L554 L555 | L556 L557 L558 L559 L560 L561 | L562 L563 L564 L565 L566 L567 | L568 L569 L570 L571 L572 L573 | L574 L575 L576 L577 L578 L579 | L580 L581 L582 L583 L584 L585 | L586 L587 L588 L589 L590 L591 | L592 L593 L594 L595 L596 L597 | L598 L599 L600 L601 L602 L603 | L604 L605 L606 L607 L608 L609 | L610 L611 L612 L613 L614 L615 | L616 L617 L618 L619 L620 L621 | L622 L623 L624 L625 L626 L627 | L628 L629 L630 L631 L632 L633 | L634 L635 L636 L637 L638 L639 | L640 L641 L642 L643 L644 L645 | L646 L647 L648 L649 L650 L651 | L652 L653 L654 L655 L656 L657 | L658 L659 L660 L661 L662 L663 | L664 L665 L666 L667 L668 L669 | L670 L671 L672 L673 L674 L675